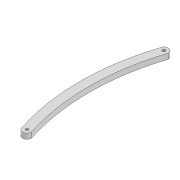
# Autodesk Inventor part: Part_4
Saved by Autodesk Inventor 2022 (Build 260153000, 153)
## iProperties
Created: 2022-04-22
Part Number: Part_4
Material: Generic
Document SubType Name: Modeling
Designer: dell
Density: 1 g/cm^3
Appearance: Default
Mass: 2.14429 g
Surface Area: 18.9003 cm^2
Volume: 2.14429 cm^3
Author: dell
Autodesk Inventor part; units mm, degrees
ref_plane "YZ Plane" through (0, 0, 0) normal (1, 0, 0) x (0, 1, 0)
ref_plane "XZ Plane" through (0, 0, 0) normal (0, 1, 0) x (-1, 0, 0)
ref_plane "XY Plane" through (0, 0, 0) normal (0, 0, 1) x (1, 0, 0)
sketch "Sketch1" plane through (0, 0, 0) normal (0, 1, 0) x (-1, 0, 0)
  line L0 (0, 0) -> (0, -153.584) construction
  line L1 (5, 0) -> (5, -153.584)
  line L2 (-5, -153.584) -> (-5, 0)
  arc A0 (5, 0) -> (-5, 0) centre (0, 0) ccw
  arc A1 (-5, -153.584) -> (5, -153.584) centre (0, -153.584) ccw
  circle A2 centre (0, 0) radius 1.65
  circle A3 centre (0, -153.584) radius 1.65
  arc A4 (-5, -153.584) -> (-5, 0) centre (-242.9138, -76.792) ccw
  arc A5 (5, -153.584) -> (5, 0) centre (-232.9138, -76.792) ccw
  point P0 (0, -76.792)
  dimension "d0" = 3.3
  dimension "d1" = 3.3
  dimension "d2" = 10
  dimension "d3" = 153.584
  dimension "d12" = 250
  dimension "d13" = 250
  constraints: 8 end point, 8 point on circle, 6 centre point, 4 tangent, 2 coincident, 1 midpoint, 1 parallel, 1 vertical
  measures "d0" diameter of A2
  measures "d1" diameter of A3
  measures "d2" distance between parallel lines of L2 L1
  measures "d3" distance of L0.end L0.start
  measures "d12" radius of A4
  measures "d13" radius of A5
extrude "Extrusion1" add sketch "Sketch1" along normal blind 6 contours A5 L1 A4 | L1 A4 A0 | A1 A4 L1
body "Solid1"
